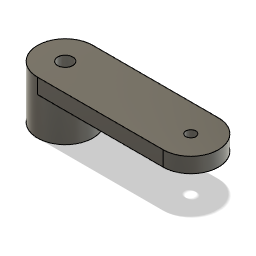
mecaniqueStatuette v11 (Autodesk Fusion 360 archive; units mm, degrees)
design "BrasServo"
Autodesk Fusion 360 part; units mm, degrees
sketch "Sketch1" plane through (0, 0, 0) normal (0, 1, 0) x (1, 0, 0)
  circle A0 centre (0, 0) radius 2.75
  circle A1 centre (0, 0) radius 5.5
  line L0 (0, 0) -> (0, 5.5) construction
  line L1 (0, 0) -> (0, -5.5) construction
  line L2 (0, 5.5) -> (30.5, 5.5)
  line L3 (30.5, 5.5) -> (30.5, -5.5)
  line L4 (30.5, -5.5) -> (0, -5.5)
  line L5 (0, -5.5) -> (0, 5.5)
  line L6 (0, 0) -> (25, 0) construction
  circle A2 centre (25, 0) radius 1
  circle A3 centre (25, 0) radius 5.5
  circle A4 centre (0, 0) radius 1.5
  dimension "d1" = 5.5
  dimension "d2" = 11
  dimension "d4" = 11
  dimension "d5" = 25
  dimension "d6" = 2
  dimension "d11" = 3
  constraint coincident A0.centre A1.centre
  constraint concentric A0 A1
  constraint coincident A1 L0.end
  constraint vertical L0
  constraint coincident A1 L1.end
  constraint parallel L0 L1
  constraint horizontal L2
  constraint vertical L3
  constraint horizontal L4
  constraint vertical L5
  constraint perpendicular L5 L6
  constraint coincident L6.end A2.centre
  constraint concentric A2 A3
  constraint tangent L2 A3
  constraint tangent L3 A3
  constraint concentric A1 A4
  measures "d1" diameter of A0
  measures "d2" diameter of A1
  measures "d4" distance of L0.end L1.end
  measures "d5" distance of A0.centre L6.end
  measures "d6" diameter of A2
  measures "d11" diameter of A4
extrude "Extrude1" add sketch "Sketch1" along normal blind 3 contours A0 A1 L5 | A0 A1 L5 | A1 L2 L4 A3 | A3
extrude "Extrude2" add sketch "Sketch1" against normal blind 7.5 contours A0 A1 L5 | A0 A1 L5
extrude "Extrude4" add sketch "Sketch1" along normal blind 3 and the other way blind 4.5 contours A0 L5 A4 | A0 L5 A4
named bodies: "BrasServo"
